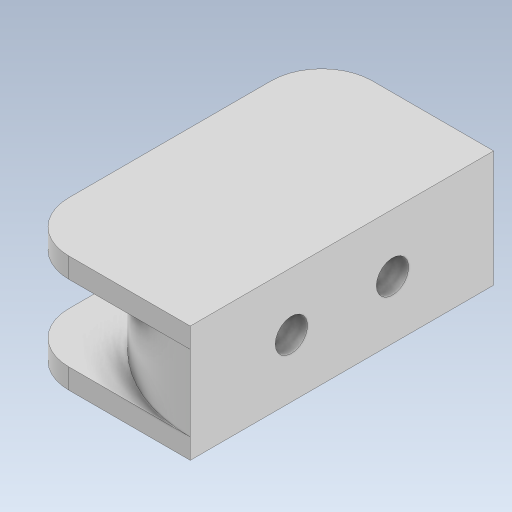
# Autodesk Inventor part: Katrol Lifter
Saved by Autodesk Inventor 2023.5 (Build 275446000, 446)
## iProperties
Created: 2025-10-19
Part Number: Katrol Lifter
Material: Generic
Document SubType Name: Modeling
Designer: Guntur
Density: 1 g/cm^3
Appearance: Default
Author: Guntur
## iProperties of the stored document Katrol Lifter_3DPrint.ipt
Created: 2025-10-20
Part Number: Katrol Lifter_3DPrint
Material: Generic
Document SubType Name: Modeling
Designer: Guntur
Density: 1 g/cm^3
Appearance: Default
Author: Guntur
Autodesk Inventor part; units mm, degrees
ref_plane "YZ Plane" through (0, 0, 0) normal (1, 0, 0) x (0, 1, 0)
ref_plane "XZ Plane" through (0, 0, 0) normal (0, 1, 0) x (-1, 0, 0)
sketch "Sketch1" plane through (0, 0, 0) normal (0, 1, 0) x (-1, 0, 0)
  circle A0 centre (0, 0) radius 15
  line L0 (0, -15) -> (0, 15)
  dimension "d0" = 30
  constraints: 2 end point, 1 coincident, 3 other
extrude "Extrusion2" add sketch "Sketch1" along normal mid plane 11.5 contours A0 L0 picked at (3.1174, 3.9092)
sketch "Sketch2" plane through (0, 5.75, 0) normal (0, 1, 0) x (1, 0, 0)
  line L0 (0, -15) -> (0, 15) projected
  line L1 (0, -15) -> (-17, -15)
  line L2 (-17, -15) -> (-17, 15)
  line L3 (-17, 15) -> (0, 15)
  line L4 (0, 15) -> (0, -15)
  point P0 (0, 0)
  constraints: 8 end point, 2 parallel, 1 horizontal, 1 perpendicular
extrude "Extrusion3" add sketch "Sketch2" against normal blind 2
sketch "Sketch3" plane through (0, -5.75, 0) normal (0, -1, 0) x (1, 0, 0)
  arc A0 (0, 15) -> (0, -15) centre (0, 0) ccw projected
  line L0 (-17, 15) -> (-17, -15) projected
  line L1 (0, -15) -> (-17, -15)
  line L2 (-17, -15) -> (-17, 15)
  line L3 (-17, 15) -> (0, 15)
  line L4 (0, 15) -> (0, -15)
  constraints: 8 end point, 2 parallel, 1 horizontal, 1 perpendicular
extrude "Extrusion4" add sketch "Sketch3" against normal blind 2 contours A0 L1 L0 L3
ref_plane "Work Plane1" through (-15, 0, 0) normal (-1, 0, 0) x (0, 0, 1)
sketch "Sketch5" plane through (-15, 0, 0) normal (-1, 0, 0) x (0, 0, 1)
  circle A0 centre (-5, 0) radius 1.6
  line L0 (-15, 3.75) -> (-15, -3.75) projected
  circle A1 centre (5, 0) radius 1.6
  line L1 (15, -3.75) -> (15, 3.75) projected
  circle A2 centre (-5, 0) radius 2.75
  circle A3 centre (5, 0) radius 2.75
  point P0 (0, 0)
  dimension "d10" = 3.2
  dimension "d11" = 10
  dimension "d12" = 3.2
  dimension "d13" = 10
  dimension "d14" = 5.5
  dimension "d15" = 5.5
  constraints: 4 centre point, 2 coincident
  measures "d10" diameter of A0
  measures "d11" distance from line of L0 A0.centre
  measures "d12" diameter of A1
  measures "d13" distance from line of L1 A1.centre
  measures "d14" diameter of A2
  measures "d15" diameter of A3
extrude "Extrusion5" cut sketch "Sketch5" against normal blind 15 contours A0 | A1
extrude "Extrusion6" cut sketch "Sketch5" against normal blind 9
fillet "Fillet1" radius 5 4 edges at (-17, 4.75, -15) (-17, 4.75, 15) (-17, -4.75, 15) (-17, -4.75, -15)
body "Solid2"
